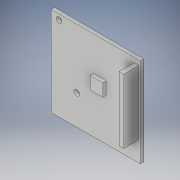
# Autodesk Inventor part: Part1
Saved by Autodesk Inventor 2017 (Build 210142000, 142)
## iProperties
Created: 2016-10-27
Part Number: Part1
Material: Generic
Document SubType Name: Modeling
Designer: cad
Density: 1 g/cm^3
Appearance: Default
Author: cad
Autodesk Inventor part; units mm, degrees
ref_plane "YZ Plane" through (0, 0, 0) normal (1, 0, 0) x (0, 1, 0)
ref_plane "XZ Plane" through (0, 0, 0) normal (0, 1, 0) x (-1, 0, 0)
ref_plane "XY Plane" through (0, 0, 0) normal (0, 0, 1) x (1, 0, 0)
sketch "Sketch1" plane through (0, 0, 0) normal (0, 0, 1) x (1, 0, 0)
  point P0 (0, 0)
sketch "Sketch2" plane through (0, 0, 0) normal (0, 0, 1) x (1, 0, 0)
  line L0 (0, 0) -> (50, 0)
  line L1 (50, 0) -> (50, 50)
  line L2 (50, 50) -> (0, 50)
  circle A0 centre (4.4, 47) radius 1.6
  circle A1 centre (14.3, 16.7) radius 1.6
  line L3 (0, 50) -> (3, 50) construction
  circle A2 centre (41.9, 12.5) radius 1.6
  line L4 (30.9, 23.8) -> (30.9, 30.8)
  line L5 (30.9, 30.8) -> (23.9, 30.8)
  line L6 (23.9, 30.8) -> (23.9, 23.8)
  line L7 (23.9, 23.8) -> (30.9, 23.8)
  line L8 (0, 50) -> (0, 0)
  dimension "d0" = 50
  dimension "d1" = 50
  dimension "d2" = 3.2
  dimension "d3" = 3.2
  dimension "d23" = 3.2
  dimension "d28" = 7
  dimension "d29" = 7
  dimension "d30" = 7
  dimension "d31" = 90
  constraints: 18 end point, 3 centre point, 3 horizontal, 3 perpendicular, 1 parallel, 1 vertical
  measures "d0" distance of L2.end L1.end
  measures "d1" distance of L1.end L0.end
  measures "d2" diameter of A0
  measures "d3" diameter of A1
  measures "d23" diameter of A2
  measures "d28" distance of L4.start L4.end
  measures "d29" distance of L4.end L5.end
  measures "d30" distance of L5.end L6.end
  measures "d31" angle of L6 L5
sketch "Sketch7" plane through (0, 0, 0) normal (0, 0, 1) x (1, 0, 0)
  line L0 (30.9, 23.8) -> (30.9, 30.8)
  line L1 (30.9, 30.8) -> (23.9, 30.8)
  line L2 (23.9, 30.8) -> (23.9, 23.8)
  line L3 (23.9, 23.8) -> (30.9, 23.8)
  point P0 (0, 0)
  dimension "d32" = 7
  dimension "d33" = 7
  dimension "d34" = 7
  dimension "d35" = 90
  constraints: 8 end point, 2 perpendicular, 1 horizontal
  measures "d32" distance of L0.start L1.start
  measures "d33" distance of L1.start L1.end
  measures "d34" distance of L1.end L3.start
  measures "d35" angle of L2 L1
extrude "Extrusion4" add sketch "Sketch2" against normal blind 2 contours L8 L2 L1 L0 | L7 L6 L5 L4
extrude "Extrusion5" add sketch "Sketch7" along normal blind 2 separate body
sketch "Sketch8" plane through (0, 0, 0) normal (0, 0, 1) x (1, 0, 0)
  line L0 (46.63, 47.4) -> (46.63, 11.24)
  line L1 (46.63, 11.24) -> (49.17, 11.24)
  line L2 (49.17, 11.24) -> (49.17, 47.4)
  line L3 (46.63, 47.4) -> (49.17, 47.4)
  point P0 (0, 0)
  constraints: 8 end point, 1 horizontal, 1 perpendicular
extrude "Extrusion6" add sketch "Sketch8" along normal blind 8.5 separate body
body "Solid2"
body "Solid3"
body "Solid4"
